Autodesk Inventor part; units mm, degrees
(part 5 of 5)
  line L348 (1.6512, 10.8975) -> (1.3983, 10.8975)
  line L349 (1.3983, 10.8975) -> (1.3983, 8.8084)
  line L350 (1.3983, 8.8084) -> (1.6512, 8.8084)
  line L351 (0.891, 9.7257) -> (0.0985, 9.7257)
  line L352 (1.1098, 8.9008) -> (1.1098, 9.1763)
  line L353 (1.1098, 9.1763) -> (1.0953, 9.1763)
  line L354 (0.0985, 9.5329) -> (1.1374, 9.5329)
  line L355 (1.1374, 9.5329) -> (1.1374, 9.6706)
  line L356 (-0.673, 10.0402) -> (-0.673, 9.1731)
  line L357 (-0.4201, 8.8084) -> (-0.4201, 10.8975)
  line L358 (-0.4201, 10.8975) -> (-0.673, 10.8975)
  line L359 (-0.673, 10.8975) -> (-0.673, 10.2492)
  line L360 (-0.673, 8.9607) -> (-0.673, 8.8084)
  line L361 (-0.673, 8.8084) -> (-0.4201, 8.8084)
  line L362 (-3.0409, 9.5944) -> (-3.0409, 9.1779)
  line L363 (-3.0409, 8.9672) -> (-3.0409, 8.8084)
  line L364 (-3.0409, 8.8084) -> (-2.7881, 8.8084)
  line L365 (-2.7881, 8.8084) -> (-2.7881, 9.8343)
  line L366 (-3.8626, 10.2768) -> (-3.8626, 10.0191)
  line L367 (-3.8626, 10.0191) -> (-3.848, 10.0191)
  line L368 (-3.0409, 9.844) -> (-3.0409, 9.7954)
  line L369 (-5.4996, 10.5588) -> (-5.4996, 10.8214)
  line L370 (-5.4996, 10.8214) -> (-5.7864, 10.8214)
  line L371 (-5.7864, 10.8214) -> (-5.7864, 10.5588)
  line L372 (-5.7864, 10.5588) -> (-5.4996, 10.5588)
  line L373 (-6.13, 8.8084) -> (-6.13, 9.7825)
  line L374 (-7.0555, 10.1423) -> (-7.0555, 10.3092)
  line L375 (-7.0555, 10.3092) -> (-7.3083, 10.3092)
  line L376 (-7.3083, 10.3092) -> (-7.3083, 8.8084)
  line L377 (-7.3083, 8.8084) -> (-7.0555, 8.8084)
  line L378 (-7.0555, 8.8084) -> (-7.0555, 9.9299)
  line L379 (-6.3829, 9.6641) -> (-6.3829, 8.8084)
  line L380 (-6.3829, 8.8084) -> (-6.13, 8.8084)
  line L381 (-7.9161, 9.5944) -> (-7.9161, 9.1779)
  line L382 (-7.9161, 8.9672) -> (-7.9161, 8.8084)
  line L383 (-7.9161, 8.8084) -> (-7.6633, 8.8084)
  line L384 (-7.6633, 8.8084) -> (-7.6633, 9.8343)
  line L385 (-8.7378, 10.2768) -> (-8.7378, 10.0191)
  line L386 (-8.7378, 10.0191) -> (-8.7232, 10.0191)
  line L387 (-7.9161, 9.844) -> (-7.9161, 9.7954)
  line L388 (-10.2516, 8.8927) -> (-10.2516, 9.1763)
  line L389 (-10.2516, 9.1763) -> (-10.2662, 9.1763)
  line L390 (-10.2662, 9.9445) -> (-10.2516, 9.9445)
  line L391 (-10.2516, 9.9445) -> (-10.2516, 10.2282)
  line L392 (-11.7929, 9.7257) -> (-12.5855, 9.7257)
  line L393 (-11.5741, 8.9008) -> (-11.5741, 9.1763)
  line L394 (-11.5741, 9.1763) -> (-11.5887, 9.1763)
  line L395 (-12.5855, 9.5329) -> (-11.5466, 9.5329)
  line L396 (-11.5466, 9.5329) -> (-11.5466, 9.6706)
  line L397 (-16.2597, 10.5588) -> (-16.2597, 10.8214)
  line L398 (-16.2597, 10.8214) -> (-16.5466, 10.8214)
  line L399 (-16.5466, 10.8214) -> (-16.5466, 10.5588)
  line L400 (-16.5466, 10.5588) -> (-16.2597, 10.5588)
  line L401 (-20.5936, 8.8214) -> (-20.5936, 9.0483)
  line L402 (-20.5936, 9.0483) -> (-20.6081, 9.0483)
  line L403 (-21.0587, 9.3854) -> (-21.0587, 10.1001)
  line L404 (-21.0587, 10.1001) -> (-20.5936, 10.1001)
  line L405 (-20.5936, 10.1001) -> (-20.5936, 10.3092)
  line L406 (-20.5936, 10.3092) -> (-21.0587, 10.3092)
  line L407 (-21.0587, 10.3092) -> (-21.0587, 10.7403)
  line L408 (-21.0587, 10.7403) -> (-21.3116, 10.7403)
  line L409 (-21.3116, 10.7403) -> (-21.3116, 10.3092)
  line L410 (-21.3116, 10.3092) -> (-21.4817, 10.3092)
  line L411 (-21.4817, 10.3092) -> (-21.4817, 10.1001)
  line L412 (-21.4817, 10.1001) -> (-21.3116, 10.1001)
  line L413 (-21.3116, 10.1001) -> (-21.3116, 9.2687)
  line L414 (-26.9047, 10.0385) -> (-26.9047, 10.3011)
  line L415 (-27.4477, 10.0855) -> (-27.4477, 10.3092)
  line L416 (-27.4477, 10.3092) -> (-27.7005, 10.3092)
  line L417 (-27.7005, 10.3092) -> (-27.7005, 8.8084)
  line L418 (-27.7005, 8.8084) -> (-27.4477, 8.8084)
  line L419 (-27.4477, 8.8084) -> (-27.4477, 9.8732)
  line L420 (-26.9177, 10.0385) -> (-26.9047, 10.0385)
  line L421 (-28.7508, 9.7808) -> (-28.9323, 9.7808)
  line L422 (-28.9323, 9.7808) -> (-28.9323, 10.5782)
  line L423 (-28.9323, 10.5782) -> (-28.7119, 10.5782)
  line L424 (-28.6957, 10.8084) -> (-29.1981, 10.8084)
  line L425 (-29.1981, 10.8084) -> (-29.1981, 8.8084)
  line L426 (-29.1981, 8.8084) -> (-28.9323, 8.8084)
  line L427 (-28.9323, 8.8084) -> (-28.9323, 9.5539)
  line L428 (-28.9323, 9.5539) -> (-28.707, 9.5539)
  line L429 (-24.3148, 10.0402) -> (-24.3148, 9.2152)
  line L430 (-25.1624, 8.5685) -> (-25.1754, 8.5685)
  line L431 (-25.1754, 8.5685) -> (-25.1754, 8.306)
  line L432 (-24.062, 8.9802) -> (-24.062, 10.3092)
  line L433 (-24.062, 10.3092) -> (-24.3002, 10.3092)
  line L434 (-24.3002, 10.3092) -> (-24.3148, 10.246)
  line L435 (-24.3148, 9.0077) -> (-24.3148, 8.8765)
  line L436 (-22.7508, 9.7257) -> (-23.5433, 9.7257)
  line L437 (-22.532, 8.9008) -> (-22.532, 9.1763)
  line L438 (-22.532, 9.1763) -> (-22.5466, 9.1763)
  line L439 (-23.5433, 9.5329) -> (-22.5044, 9.5329)
  line L440 (-22.5044, 9.5329) -> (-22.5044, 9.6706)
  line L441 (-21.5141, 8.8214) -> (-21.5141, 9.0483)
  line L442 (-21.5141, 9.0483) -> (-21.5287, 9.0483)
  line L443 (-21.9793, 9.3854) -> (-21.9793, 10.1001)
  line L444 (-21.9793, 10.1001) -> (-21.5141, 10.1001)
  line L445 (-21.5141, 10.1001) -> (-21.5141, 10.3092)
  line L446 (-21.5141, 10.3092) -> (-21.9793, 10.3092)
  line L447 (-21.9793, 10.3092) -> (-21.9793, 10.7403)
  line L448 (-21.9793, 10.7403) -> (-22.2321, 10.7403)
  line L449 (-22.2321, 10.7403) -> (-22.2321, 10.3092)
  line L450 (-22.2321, 10.3092) -> (-22.4023, 10.3092)
  line L451 (-22.4023, 10.3092) -> (-22.4023, 10.1001)
  line L452 (-22.4023, 10.1001) -> (-22.2321, 10.1001)
  line L453 (-22.2321, 10.1001) -> (-22.2321, 9.2687)
  line L454 (-17.1543, 10.0402) -> (-17.1543, 9.1731)
  line L455 (-16.9015, 8.8084) -> (-16.9015, 10.8975)
  line L456 (-16.9015, 10.8975) -> (-17.1543, 10.8975)
  line L457 (-17.1543, 10.8975) -> (-17.1543, 10.2492)
  line L458 (-17.1543, 8.9607) -> (-17.1543, 8.8084)
  line L459 (-17.1543, 8.8084) -> (-16.9015, 8.8084)
  line L460 (-16.2775, 8.8084) -> (-16.2775, 10.3092)
  line L461 (-16.2775, 10.3092) -> (-16.5304, 10.3092)
  line L462 (-16.5304, 10.3092) -> (-16.5304, 8.8084)
  line L463 (-16.5304, 8.8084) -> (-16.2775, 8.8084)
  line L464 (-13.3456, 8.8084) -> (-13.0928, 8.8084)
  line L465 (-13.0928, 8.8084) -> (-13.0928, 9.797)
  line L466 (-14.7945, 10.1439) -> (-14.7945, 10.3092)
  line L467 (-14.7945, 10.3092) -> (-15.0474, 10.3092)
  line L468 (-15.0474, 10.3092) -> (-15.0474, 8.8084)
  line L469 (-15.0474, 8.8084) -> (-14.7945, 8.8084)
  line L470 (-14.7945, 8.8084) -> (-14.7945, 9.9299)
  line L471 (-14.1965, 9.6771) -> (-14.1965, 8.8084)
  line L472 (-14.1965, 8.8084) -> (-13.9436, 8.8084)
  line L473 (-13.9436, 8.8084) -> (-13.9436, 9.797)
  line L474 (-13.3456, 9.6771) -> (-13.3456, 8.8084)
  line L475 (-8.9825, 8.8927) -> (-8.9825, 9.1763)
  line L476 (-8.9825, 9.1763) -> (-8.9971, 9.1763)
  line L477 (-8.9971, 9.9445) -> (-8.9825, 9.9445)
  line L478 (-8.9825, 9.9445) -> (-8.9825, 10.2282)
  line L479 (-5.5174, 8.8084) -> (-5.5174, 10.3092)
  line L480 (-5.5174, 10.3092) -> (-5.7702, 10.3092)
  line L481 (-5.7702, 10.3092) -> (-5.7702, 8.8084)
  line L482 (-5.7702, 8.8084) -> (-5.5174, 8.8084)
  line L483 (-4.1073, 8.8927) -> (-4.1073, 9.1763)
  line L484 (-4.1073, 9.1763) -> (-4.1219, 9.1763)
  line L485 (-4.1219, 9.9445) -> (-4.1073, 9.9445)
  line L486 (-4.1073, 9.9445) -> (-4.1073, 10.2282)
  line L487 (2.28, 8.8084) -> (2.28, 10.8975)
  line L488 (2.28, 10.8975) -> (2.0272, 10.8975)
  line L489 (2.0272, 10.8975) -> (2.0272, 8.8084)
  line L490 (2.0272, 8.8084) -> (2.28, 8.8084)
  line L491 (6.5847, 8.8084) -> (6.5847, 10.3092)
  line L492 (6.5847, 10.3092) -> (6.3319, 10.3092)
  line L493 (6.3319, 10.3092) -> (6.3319, 8.8084)
  line L494 (6.3319, 8.8084) -> (6.5847, 8.8084)
  line L495 (7.2087, 9.079) -> (7.2087, 9.9397)
  line L496 (7.2087, 10.152) -> (7.2087, 10.8975)
  line L497 (7.2087, 10.8975) -> (6.9559, 10.8975)
  line L498 (6.9559, 10.8975) -> (6.9559, 8.8084)
  line L499 (6.9559, 8.8084) -> (7.1925, 8.8084)
  line L500 (7.1925, 8.8084) -> (7.2087, 8.8781)
  line L501 (9.2719, 10.0385) -> (9.2719, 10.3011)
  line L502 (8.729, 10.0855) -> (8.729, 10.3092)
  line L503 (8.729, 10.3092) -> (8.4761, 10.3092)
  line L504 (8.4761, 10.3092) -> (8.4761, 8.8084)
  line L505 (8.4761, 8.8084) -> (8.729, 8.8084)
  line L506 (8.729, 8.8084) -> (8.729, 9.8732)
  line L507 (9.2589, 10.0385) -> (9.2719, 10.0385)
  line L508 (12.3919, 8.8084) -> (12.3919, 10.3092)
  line L509 (12.3919, 10.3092) -> (12.139, 10.3092)
  line L510 (12.139, 10.3092) -> (12.139, 8.8084)
  line L511 (12.139, 8.8084) -> (12.3919, 8.8084)
  line L512 (15.434, 8.8084) -> (15.434, 9.7825)
  line L513 (14.5085, 10.1423) -> (14.5085, 10.3092)
  line L514 (14.5085, 10.3092) -> (14.2557, 10.3092)
  line L515 (14.2557, 10.3092) -> (14.2557, 8.8084)
  line L516 (14.2557, 8.8084) -> (14.5085, 8.8084)
  line L517 (14.5085, 8.8084) -> (14.5085, 9.9299)
  line L518 (15.1812, 9.6641) -> (15.1812, 8.8084)
  line L519 (15.1812, 8.8084) -> (15.434, 8.8084)
  line L520 (16.0645, 10.5588) -> (16.0645, 10.8214)
  line L521 (16.0645, 10.8214) -> (15.7776, 10.8214)
  line L522 (15.7776, 10.8214) -> (15.7776, 10.5588)
  line L523 (15.7776, 10.5588) -> (16.0645, 10.5588)
  line L524 (21.374, 8.8084) -> (21.374, 9.0126)
  line L525 (21.374, 9.0126) -> (21.0191, 9.0126)
  line L526 (21.0191, 9.0126) -> (21.0191, 10.8149)
  line L527 (21.0191, 10.8149) -> (20.8116, 10.8149)
  line L528 (20.3983, 10.5361) -> (20.3983, 10.353)
  line L529 (20.3983, 10.353) -> (20.7614, 10.353)
  line L530 (20.7614, 10.353) -> (20.7614, 9.0126)
  line L531 (20.7614, 9.0126) -> (20.3983, 9.0126)
  line L532 (20.3983, 9.0126) -> (20.3983, 8.8084)
  line L533 (20.3983, 8.8084) -> (21.374, 8.8084)
  line L534 (25.528, 8.8084) -> (25.528, 9.0402)
  line L535 (25.528, 9.0402) -> (24.5458, 9.0402)
  line L536 (24.3367, 10.7306) -> (24.3367, 10.4453)
  line L537 (24.3367, 10.4453) -> (24.3513, 10.4453)
  line L538 (24.2946, 9.092) -> (24.2946, 8.8084)
  line L539 (24.2946, 8.8084) -> (25.528, 8.8084)
  line L540 (-26.7605, 6.3015) -> (-26.7605, 5.885)
  line L541 (-26.7605, 5.6743) -> (-26.7605, 5.5154)
  line L542 (-26.7605, 5.5154) -> (-26.5077, 5.5154)
  line L543 (-26.5077, 5.5154) -> (-26.5077, 6.5414)
  line L544 (-27.5822, 6.9838) -> (-27.5822, 6.7261)
  line L545 (-27.5822, 6.7261) -> (-27.5676, 6.7261)
  line L546 (-26.7605, 6.5511) -> (-26.7605, 6.5025)
  line L547 (-24.9744, 5.5154) -> (-24.9744, 6.4895)
  line L548 (-25.8999, 6.8493) -> (-25.8999, 7.0162)
  line L549 (-25.8999, 7.0162) -> (-26.1527, 7.0162)
  line L550 (-26.1527, 7.0162) -> (-26.1527, 5.5154)
  line L551 (-26.1527, 5.5154) -> (-25.8999, 5.5154)
  line L552 (-25.8999, 5.5154) -> (-25.8999, 6.637)
  line L553 (-25.2273, 6.3712) -> (-25.2273, 5.5154)
  line L554 (-25.2273, 5.5154) -> (-24.9744, 5.5154)
  line L555 (-20.0976, 6.7472) -> (-20.0976, 5.8801)
  line L556 (-19.8448, 5.5154) -> (-19.8448, 7.6046)
  line L557 (-19.8448, 7.6046) -> (-20.0976, 7.6046)
  line L558 (-20.0976, 7.6046) -> (-20.0976, 6.9563)
  line L559 (-20.0976, 5.6678) -> (-20.0976, 5.5154)
  line L560 (-20.0976, 5.5154) -> (-19.8448, 5.5154)
  line L561 (-19.2208, 5.5154) -> (-19.2208, 7.0162)
  line L562 (-19.2208, 7.0162) -> (-19.4736, 7.0162)
  line L563 (-19.4736, 7.0162) -> (-19.4736, 5.5154)
  line L564 (-19.4736, 5.5154) -> (-19.2208, 5.5154)
  line L565 (-17.7378, 5.7958) -> (-17.7378, 6.6483)
  line L566 (-17.7378, 6.859) -> (-17.7378, 7.0162)
  line L567 (-17.7378, 7.0162) -> (-17.9906, 7.0162)
  line L568 (-17.9906, 7.0162) -> (-17.9906, 4.9628)
  line L569 (-17.9906, 4.9628) -> (-17.7378, 4.9628)
  line L570 (-17.7378, 4.9628) -> (-17.7378, 5.5916)
  line L571 (-15.6746, 6.7456) -> (-15.6746, 7.0081)
  line L572 (-16.2175, 6.7926) -> (-16.2175, 7.0162)
  line L573 (-16.2175, 7.0162) -> (-16.4704, 7.0162)
  line L574 (-16.4704, 7.0162) -> (-16.4704, 5.5154)
  line L575 (-16.4704, 5.5154) -> (-16.2175, 5.5154)
  line L576 (-16.2175, 5.5154) -> (-16.2175, 6.5803)
  line L577 (-15.6876, 6.7456) -> (-15.6746, 6.7456)
  line L578 (-11.7799, 6.3015) -> (-11.7799, 5.885)
  line L579 (-11.7799, 5.6743) -> (-11.7799, 5.5154)
  line L580 (-11.7799, 5.5154) -> (-11.5271, 5.5154)
  line L581 (-11.5271, 5.5154) -> (-11.5271, 6.5414)
  line L582 (-12.6017, 6.9838) -> (-12.6017, 6.7261)
  line L583 (-12.6017, 6.7261) -> (-12.5871, 6.7261)
  line L584 (-11.7799, 6.5511) -> (-11.7799, 6.5025)
  line L585 (-10.0603, 5.7958) -> (-10.0603, 6.6483)
  line L586 (-10.0603, 6.859) -> (-10.0603, 7.0162)
  line L587 (-10.0603, 7.0162) -> (-10.3132, 7.0162)
  line L588 (-10.3132, 7.0162) -> (-10.3132, 4.9628)
  line L589 (-10.3132, 4.9628) -> (-10.0603, 4.9628)
  line L590 (-10.0603, 4.9628) -> (-10.0603, 5.5916)
  line L591 (-7.848, 6.4328) -> (-8.6406, 6.4328)
  line L592 (-7.6292, 5.6078) -> (-7.6292, 5.8833)
  line L593 (-7.6292, 5.8833) -> (-7.6438, 5.8833)
  line L594 (-8.6406, 6.2399) -> (-7.6017, 6.2399)
  line L595 (-7.6017, 6.2399) -> (-7.6017, 6.3777)
  line L596 (-6.5498, 6.7456) -> (-6.5498, 7.0081)
  line L597 (-7.0928, 6.7926) -> (-7.0928, 7.0162)
  line L598 (-7.0928, 7.0162) -> (-7.3456, 7.0162)
  line L599 (-7.3456, 7.0162) -> (-7.3456, 5.5154)
  line L600 (-7.3456, 5.5154) -> (-7.0928, 5.5154)
  line L601 (-7.0928, 5.5154) -> (-7.0928, 6.5803)
  line L602 (-6.5628, 6.7456) -> (-6.5498, 6.7456)
  line L603 (-0.9582, 5.5284) -> (-0.9582, 5.7553)
  line L604 (-0.9582, 5.7553) -> (-0.9728, 5.7553)
  line L605 (-1.4234, 6.0924) -> (-1.4234, 6.8072)
  line L606 (-1.4234, 6.8072) -> (-0.9582, 6.8072)
  line L607 (-0.9582, 6.8072) -> (-0.9582, 7.0162)
  line L608 (-0.9582, 7.0162) -> (-1.4234, 7.0162)
  line L609 (-1.4234, 7.0162) -> (-1.4234, 7.4474)
  line L610 (-1.4234, 7.4474) -> (-1.6762, 7.4474)
  line L611 (-1.6762, 7.4474) -> (-1.6762, 7.0162)
  line L612 (-1.6762, 7.0162) -> (-1.8464, 7.0162)
  line L613 (-1.8464, 7.0162) -> (-1.8464, 6.8072)
  line L614 (-1.8464, 6.8072) -> (-1.6762, 6.8072)
  line L615 (-1.6762, 6.8072) -> (-1.6762, 5.9757)
  line L616 (2.6577, 6.4328) -> (1.8651, 6.4328)
  line L617 (2.8765, 5.6078) -> (2.8765, 5.8833)
  line L618 (2.8765, 5.8833) -> (2.8619, 5.8833)
  line L619 (1.8651, 6.2399) -> (2.904, 6.2399)
  line L620 (2.904, 6.2399) -> (2.904, 6.3777)
  line L621 (4.5069, 5.7456) -> (4.3043, 5.7456)
  line L622 (4.3043, 5.7456) -> (4.3043, 7.2853)
  line L623 (4.3043, 7.2853) -> (4.5069, 7.2853)
  line L624 (4.494, 7.5154) -> (4.0385, 7.5154)
  line L625 (4.0385, 7.5154) -> (4.0385, 5.5154)
  line L626 (4.0385, 5.5154) -> (4.4988, 5.5154)
  line L627 (7.3076, 5.6516) -> (7.3076, 5.9692)
  line L628 (7.3076, 5.9692) -> (7.2881, 5.9692)
  line L629 (7.2865, 7.0616) -> (7.3076, 7.0616)
  line L630 (7.3076, 7.0616) -> (7.3076, 7.3825)
  line L631 (-24.2727, 2.2225) -> (-24.2727, 3.7233)
  line L632 (-24.2727, 3.7233) -> (-24.5255, 3.7233)
  line L633 (-24.5255, 3.7233) -> (-24.5255, 2.6017)
  line L634 (-25.1981, 2.8675) -> (-25.1981, 3.7233)
  line L635 (-25.1981, 3.7233) -> (-25.4509, 3.7233)
  line L636 (-25.4509, 3.7233) -> (-25.4509, 2.7492)
  line L637 (-24.5255, 2.3878) -> (-24.5255, 2.2225)
  line L638 (-24.5255, 2.2225) -> (-24.2727, 2.2225)
  line L639 (-22.0782, 3.0086) -> (-22.0782, 2.592)
  line L640 (-22.0782, 2.3813) -> (-22.0782, 2.2225)
  line L641 (-22.0782, 2.2225) -> (-21.8253, 2.2225)
  line L642 (-21.8253, 2.2225) -> (-21.8253, 3.2484)
  line L643 (-22.8999, 3.6909) -> (-22.8999, 3.4332)
  line L644 (-22.8999, 3.4332) -> (-22.8853, 3.4332)
  line L645 (-22.0782, 3.2581) -> (-22.0782, 3.2095)
  line L646 (-19.7103, 3.4543) -> (-19.7103, 2.5872)
  line L647 (-19.4574, 2.2225) -> (-19.4574, 4.3116)
  line L648 (-19.4574, 4.3116) -> (-19.7103, 4.3116)
  line L649 (-19.7103, 4.3116) -> (-19.7103, 3.6633)
  line L650 (-19.7103, 2.3748) -> (-19.7103, 2.2225)
  line L651 (-19.7103, 2.2225) -> (-19.4574, 2.2225)
  line L652 (-18.8334, 2.2225) -> (-18.8334, 3.7233)
  line L653 (-18.8334, 3.7233) -> (-19.0863, 3.7233)
  line L654 (-19.0863, 3.7233) -> (-19.0863, 2.2225)
  line L655 (-19.0863, 2.2225) -> (-18.8334, 2.2225)
  line L656 (-17.9987, 2.2225) -> (-17.9987, 2.605)
  line L657 (-17.9987, 2.605) -> (-18.3197, 2.605)
  line L658 (-18.3197, 2.605) -> (-18.3197, 2.2225)
  line L659 (-18.3197, 2.2225) -> (-17.9987, 2.2225)
  line L660 (-20.1495, 0.7756) -> (-20.1495, 1.0073)
  line L661 (-20.9128, 0.4806) -> (-20.9128, 0.4304)
  line L662 (-20.9128, 0.4304) -> (-21.083, 0.4304)
  line L663 (-21.083, 0.4304) -> (-21.083, 0.2213)
  line L664 (-21.083, 0.2213) -> (-20.9128, 0.2213)
  line L665 (-20.9128, 0.2213) -> (-20.9128, -1.0705)
  line L666 (-20.9128, -1.0705) -> (-20.66, -1.0705)
  line L667 (-20.66, -1.0705) -> (-20.66, 0.2213)
  line L668 (-20.66, 0.2213) -> (-20.25, 0.2213)
  line L669 (-20.25, 0.2213) -> (-20.25, 0.4304)
  line L670 (-20.25, 0.4304) -> (-20.6681, 0.4304)
  line L671 (-20.6681, 0.4304) -> (-20.6681, 0.4806)
  line L672 (-20.1624, 0.7756) -> (-20.1495, 0.7756)
  line L673 (-14.7151, -1.0705) -> (-13.4639, -1.0705)
  line L674 (-13.4639, -1.0705) -> (-13.4639, -0.8338)
  line L675 (-13.4639, -0.8338) -> (-14.4493, -0.8338)
  line L676 (-14.4493, -0.8338) -> (-14.4493, -0.0915)
  line L677 (-14.4493, -0.0915) -> (-13.5304, -0.0915)
  line L678 (-13.5304, -0.0915) -> (-13.5304, 0.1451)
  line L679 (-13.5304, 0.1451) -> (-14.4493, 0.1451)
  line L680 (-14.4493, 0.1451) -> (-14.4493, 0.6929)
  line L681 (-14.4493, 0.6929) -> (-13.4639, 0.6929)
  line L682 (-13.4639, 0.6929) -> (-13.4639, 0.9295)
  line L683 (-13.4639, 0.9295) -> (-14.7151, 0.9295)
  line L684 (-14.7151, 0.9295) -> (-14.7151, -1.0705)
  line L685 (-10.0458, -0.2844) -> (-10.0458, -0.7009)
  line L686 (-10.0458, -0.9116) -> (-10.0458, -1.0705)
  line L687 (-10.0458, -1.0705) -> (-9.7929, -1.0705)
  line L688 (-9.7929, -1.0705) -> (-9.7929, -0.0445)
  line L689 (-10.8675, 0.3979) -> (-10.8675, 0.1402)
  line L690 (-10.8675, 0.1402) -> (-10.8529, 0.1402)
  line L691 (-10.0458, -0.0348) -> (-10.0458, -0.0834)
  line L692 (-8.2597, -1.0705) -> (-8.2597, -0.0964)
  line L693 (-9.1851, 0.2634) -> (-9.1851, 0.4304)
  line L694 (-9.1851, 0.4304) -> (-9.438, 0.4304)
  line L695 (-9.438, 0.4304) -> (-9.438, -1.0705)
  line L696 (-9.438, -1.0705) -> (-9.1851, -1.0705)
  line L697 (-9.1851, -1.0705) -> (-9.1851, 0.0511)
  line L698 (-8.5125, -0.2147) -> (-8.5125, -1.0705)
  line L699 (-8.5125, -1.0705) -> (-8.2597, -1.0705)
  line L700 (-5.4266, -0.1531) -> (-6.2192, -0.1531)
  line L701 (-5.2078, -0.9781) -> (-5.2078, -0.7025)
  line L702 (-5.2078, -0.7025) -> (-5.2224, -0.7025)
  line L703 (-6.2192, -0.346) -> (-5.1803, -0.346)
  line L704 (-5.1803, -0.346) -> (-5.1803, -0.2082)
  line L705 (-4.6665, -1.0705) -> (-4.6665, 1.0187)
  line L706 (-4.6665, 1.0187) -> (-4.9193, 1.0187)
  line L707 (-4.9193, 1.0187) -> (-4.9193, -1.0705)
  line L708 (-4.9193, -1.0705) -> (-4.6665, -1.0705)
  line L709 (-22.6308, -3.1754) -> (-22.9323, -3.1754)
  line L710 (-22.9323, -3.1754) -> (-22.9323, -2.5903)
  line L711 (-22.9323, -2.5903) -> (-22.6778, -2.5903)
  line L712 (-22.7167, -4.1365) -> (-22.9323, -4.1365)
  line L713 (-22.9323, -4.1365) -> (-22.9323, -3.3974)
  line L714 (-22.9323, -3.3974) -> (-22.6308, -3.3974)
  line L715 (-22.2159, -3.2516) -> (-22.2159, -3.2418)
  line L716 (-22.6681, -2.3634) -> (-23.1981, -2.3634)
  line L717 (-23.1981, -2.3634) -> (-23.1981, -4.3634)
  line L718 (-23.1981, -4.3634) -> (-22.6244, -4.3634)
  line L719 (-15.7232, -3.5773) -> (-15.7232, -3.9939)
  line L720 (-15.7232, -4.2046) -> (-15.7232, -4.3634)
  line L721 (-15.7232, -4.3634) -> (-15.4704, -4.3634)
  line L722 (-15.4704, -4.3634) -> (-15.4704, -3.3375)
  line L723 (-16.5449, -2.895) -> (-16.5449, -3.1527)
  line L724 (-16.5449, -3.1527) -> (-16.5304, -3.1527)
  line L725 (-15.7232, -3.3277) -> (-15.7232, -3.3764)
  line L726 (-13.4137, -4.3634) -> (-13.1608, -4.3634)
  line L727 (-13.1608, -4.3634) -> (-13.1608, -3.3747)
  line L728 (-14.8626, -3.0279) -> (-14.8626, -2.8626)
  line L729 (-14.8626, -2.8626) -> (-15.1154, -2.8626)
  line L730 (-15.1154, -2.8626) -> (-15.1154, -4.3634)
  line L731 (-15.1154, -4.3634) -> (-14.8626, -4.3634)
  line L732 (-14.8626, -4.3634) -> (-14.8626, -3.2418)
  line L733 (-14.2646, -3.4947) -> (-14.2646, -4.3634)
  line L734 (-14.2646, -4.3634) -> (-14.0117, -4.3634)
  line L735 (-14.0117, -4.3634) -> (-14.0117, -3.3747)
  line L736 (-13.4137, -3.4947) -> (-13.4137, -4.3634)
  line L737 (-9.0911, -4.3504) -> (-9.0911, -4.1235)
  line L738 (-9.0911, -4.1235) -> (-9.1057, -4.1235)
  line L739 (-9.5563, -3.7864) -> (-9.5563, -3.0717)
  line L740 (-9.5563, -3.0717) -> (-9.0911, -3.0717)
  line L741 (-9.0911, -3.0717) -> (-9.0911, -2.8626)
  line L742 (-9.0911, -2.8626) -> (-9.5563, -2.8626)
  line L743 (-9.5563, -2.8626) -> (-9.5563, -2.4315)
  line L744 (-9.5563, -2.4315) -> (-9.8091, -2.4315)
  line L745 (-9.8091, -2.4315) -> (-9.8091, -2.8626)
  line L746 (-9.8091, -2.8626) -> (-9.9793, -2.8626)
  line L747 (-9.9793, -2.8626) -> (-9.9793, -3.0717)
  line L748 (-9.9793, -3.0717) -> (-9.8091, -3.0717)
  line L749 (-9.8091, -3.0717) -> (-9.8091, -3.9031)
  line L750 (-8.6292, -2.613) -> (-8.6292, -2.3504)
  line L751 (-8.6292, -2.3504) -> (-8.9161, -2.3504)
  line L752 (-8.9161, -2.3504) -> (-8.9161, -2.613)
  line L753 (-8.9161, -2.613) -> (-8.6292, -2.613)
  line L754 (-5.7248, -4.3634) -> (-5.7248, -2.8626)
  line L755 (-5.7248, -2.8626) -> (-5.9777, -2.8626)
  line L756 (-5.9777, -2.8626) -> (-5.9777, -4.3634)
  line L757 (-5.9777, -4.3634) -> (-5.7248, -4.3634)
  line L758 (-5.096, -4.3634) -> (-5.096, -2.2743)
  line L759 (-5.096, -2.2743) -> (-5.3488, -2.2743)
  line L760 (-5.3488, -2.2743) -> (-5.3488, -4.3634)
  line L761 (-5.3488, -4.3634) -> (-5.096, -4.3634)
  line L762 (-4.4493, -2.613) -> (-4.4493, -2.3504)
  line L763 (-4.4493, -2.3504) -> (-4.7362, -2.3504)
  line L764 (-4.7362, -2.3504) -> (-4.7362, -2.613)
  line L765 (-4.7362, -2.613) -> (-4.4493, -2.613)
  line L766 (-21.7475, -5.6564) -> (-22.0182, -5.6564)
  line L767 (-22.0182, -5.6564) -> (-22.5725, -7.3176)
  line L768 (-22.5725, -7.3176) -> (-23.1268, -5.6564)
  line L769 (-23.1268, -5.6564) -> (-23.412, -5.6564)
  line L770 (-23.412, -5.6564) -> (-22.7232, -7.6564)
  line L771 (-22.7232, -7.6564) -> (-22.4364, -7.6564)
  line L772 (-22.4364, -7.6564) -> (-21.7475, -5.6564)
  line L773 (-21.3002, -5.9059) -> (-21.3002, -5.6434)
  line L774 (-21.3002, -5.6434) -> (-21.5871, -5.6434)
  line L775 (-21.5871, -5.6434) -> (-21.5871, -5.9059)
  line L776 (-21.5871, -5.9059) -> (-21.3002, -5.9059)
  line L777 (-19.2921, -7.6434) -> (-19.2921, -7.4165)
  line L778 (-19.2921, -7.4165) -> (-19.3067, -7.4165)
  line L779 (-19.7573, -7.0794) -> (-19.7573, -6.3646)
  line L780 (-19.7573, -6.3646) -> (-19.2921, -6.3646)
  line L781 (-19.2921, -6.3646) -> (-19.2921, -6.1555)
  line L782 (-19.2921, -6.1555) -> (-19.7573, -6.1555)
  line L783 (-19.7573, -6.1555) -> (-19.7573, -5.7244)
  line L784 (-19.7573, -5.7244) -> (-20.0101, -5.7244)
  line L785 (-20.0101, -5.7244) -> (-20.0101, -6.1555)
  line L786 (-20.0101, -6.1555) -> (-20.1803, -6.1555)
  line L787 (-20.1803, -6.1555) -> (-20.1803, -6.3646)
  line L788 (-20.1803, -6.3646) -> (-20.0101, -6.3646)
  line L789 (-20.0101, -6.3646) -> (-20.0101, -7.1961)
  line L790 (-18.8302, -5.9059) -> (-18.8302, -5.6434)
  line L791 (-18.8302, -5.6434) -> (-19.1171, -5.6434)
  line L792 (-19.1171, -5.6434) -> (-19.1171, -5.9059)
  line L793 (-19.1171, -5.9059) -> (-18.8302, -5.9059)
  line L794 (-14.9453, -6.8703) -> (-14.9453, -7.2868)
  line L795 (-14.9453, -7.4975) -> (-14.9453, -7.6564)
  line L796 (-14.9453, -7.6564) -> (-14.6924, -7.6564)
  line L797 (-14.6924, -7.6564) -> (-14.6924, -6.6304)
  line L798 (-15.767, -6.188) -> (-15.767, -6.4457)
  line L799 (-15.767, -6.4457) -> (-15.7524, -6.4457)
  line L800 (-14.9453, -6.6207) -> (-14.9453, -6.6693)
  line L801 (-14.0846, -7.3857) -> (-14.0846, -6.5251)
  line L802 (-14.0846, -6.3128) -> (-14.0846, -5.5672)
  line L803 (-14.0846, -5.5672) -> (-14.3375, -5.5672)
  line L804 (-14.3375, -5.5672) -> (-14.3375, -7.6564)
  line L805 (-14.3375, -7.6564) -> (-14.1009, -7.6564)
  line L806 (-14.1009, -7.6564) -> (-14.0846, -7.5867)
  line L807 (-12.0214, -6.4262) -> (-12.0214, -6.1636)
  line L808 (-12.5644, -6.3792) -> (-12.5644, -6.1555)
  line L809 (-12.5644, -6.1555) -> (-12.8172, -6.1555)
  line L810 (-12.8172, -6.1555) -> (-12.8172, -7.6564)
  line L811 (-12.8172, -7.6564) -> (-12.5644, -7.6564)
  line L812 (-12.5644, -7.6564) -> (-12.5644, -6.5915)
  line L813 (-12.0344, -6.4262) -> (-12.0214, -6.4262)
  line L814 (-11.5498, -5.9059) -> (-11.5498, -5.6434)
  line L815 (-11.5498, -5.6434) -> (-11.8367, -5.6434)
  line L816 (-11.8367, -5.6434) -> (-11.8367, -5.9059)
  line L817 (-11.8367, -5.9059) -> (-11.5498, -5.9059)
  line L818 (-8.1754, -6.739) -> (-8.968, -6.739)
  line L819 (-7.9566, -7.564) -> (-7.9566, -7.2884)
  line L820 (-7.9566, -7.2884) -> (-7.9712, -7.2884)
  line L821 (-8.968, -6.9319) -> (-7.9291, -6.9319)
  line L822 (-7.9291, -6.9319) -> (-7.9291, -6.7941)
  line L823 (-19.1543, -10.865) -> (-19.1543, -10.5814)
  line L824 (-19.1543, -10.5814) -> (-19.1689, -10.5814)
  line L825 (-19.1689, -9.8132) -> (-19.1543, -9.8132)
  line L826 (-19.1543, -9.8132) -> (-19.1543, -9.5295)
  line L827 (-17.3975, -10.9493) -> (-17.3975, -9.4485)
  line L828 (-17.3975, -9.4485) -> (-17.6503, -9.4485)
  line L829 (-17.6503, -9.4485) -> (-17.6503, -10.9493)
  line L830 (-17.6503, -10.9493) -> (-17.3975, -10.9493)
  line L831 (-13.4963, -10.9493) -> (-13.4963, -10.7127)
  line L832 (-13.4963, -10.7127) -> (-14.3893, -10.7127)
  line L833 (-14.3893, -10.7127) -> (-14.3893, -8.9493)
  line L834 (-14.3893, -8.9493) -> (-14.6552, -8.9493)
  line L835 (-14.6552, -8.9493) -> (-14.6552, -10.9493)
  line L836 (-14.6552, -10.9493) -> (-13.4963, -10.9493)
  line L837 (-7.9971, -10.1632) -> (-7.9971, -10.5798)
  line L838 (-7.9971, -10.7905) -> (-7.9971, -10.9493)
  line L839 (-7.9971, -10.9493) -> (-7.7443, -10.9493)
  line L840 (-7.7443, -10.9493) -> (-7.7443, -9.9234)
  line L841 (-8.8188, -9.4809) -> (-8.8188, -9.7386)
  line L842 (-8.8188, -9.7386) -> (-8.8043, -9.7386)
  line L843 (-7.9971, -9.9136) -> (-7.9971, -9.9623)
  line L844 (-6.5936, -9.7192) -> (-6.5936, -9.4566)
  line L845 (-7.1365, -9.6722) -> (-7.1365, -9.4485)
  line L846 (-7.1365, -9.4485) -> (-7.3893, -9.4485)
  line L847 (-7.3893, -9.4485) -> (-7.3893, -10.9493)
  line L848 (-7.3893, -10.9493) -> (-7.1365, -10.9493)
  line L849 (-7.1365, -10.9493) -> (-7.1365, -9.8845)
  line L850 (-6.6065, -9.7192) -> (-6.5936, -9.7192)
  point P0 (0, 0)
  point P1 (-4.7232, -10.1989)
  point P2 (-4.3132, -9.6235)
  point P3 (-3.9047, -10.1989)
  point P4 (-4.3132, -10.7743)
  point P5 (-3.6438, -10.1989)
  point P6 (-4.3132, -9.4063)
  point P7 (-4.9842, -10.1989)
  point P8 (-4.3132, -10.9914)
  point P9 (-5.8253, -9.6381)
  point P10 (-5.8853, -10.7516)
  point P11 (-6.2402, -10.2054)
  point P12 (-5.8675, -9.4063)
  point P13 (-6.3099, -9.6154)
  point P14 (-6.5012, -10.2102)
  point P15 (-6.3472, -10.7905)
  point P16 (-5.9436, -10.9914)
  point P17 (-5.6989, -10.938)
  point P18 (-9.6584, -9.4063)
  point P19 (-9.7248, -9.6462)
  point P20 (-9.4898, -9.758)
  point P21 (-11.7054, -10.1989)
  point P22 (-11.2953, -9.6235)
  point P23 (-10.8869, -10.1989)
  point P24 (-11.2953, -10.7743)
  point P25 (-10.626, -10.1989)
  point P26 (-11.2953, -9.4063)
  point P27 (-11.9663, -10.1989)
  point P28 (-11.2953, -10.9914)
  point P29 (-12.7313, -9.6138)
  point P30 (-12.4477, -9.7305)
  point P31 (-13.0312, -9.7321)
  point P32 (-12.6552, -10.9833)
  point P33 (-12.3715, -10.9412)
  point P34 (-12.3505, -10.6965)
  point P35 (-12.6584, -10.7629)
  point P36 (-12.2824, -9.5733)
  point P37 (-12.7167, -9.4063)
  point P38 (-13.4104, -10.207)
  point P39 (-18.3278, -10.9833)
  point P40 (-18.0814, -10.9444)
  point P41 (-18.3326, -10.7629)
  point P42 (-18.767, -10.2021)
  point P43 (-18.3326, -9.6349)
  point P44 (-18.0717, -9.7013)
  point P45 (-18.3278, -9.4145)
  point P46 (-18.8334, -9.6187)
  point P47 (-19.0279, -10.2021)
  point P48 (-18.8334, -10.7905)
  point P49 (-22.6406, -10.985)
  point P50 (-22.1187, -10.8034)
  point P51 (-21.9372, -10.3788)
  point P52 (-22.3342, -9.8747)
  point P53 (-22.7443, -9.7694)
  point P54 (-23.0052, -9.4582)
  point P55 (-22.5919, -9.1438)
  point P56 (-22.6098, -8.9136)
  point P57 (-23.2824, -9.4858)
  point P58 (-23.1527, -9.8472)
  point P59 (-22.8221, -10.0239)
  point P60 (-22.4607, -10.1146)
  point P61 (-22.2143, -10.4209)
  point P62 (-22.66, -10.7548)
  point P63 (-10.6211, -6.3209)
  point P64 (-10.3375, -6.4376)
  point P65 (-10.921, -6.4392)
  point P66 (-10.5449, -7.6904)
  point P67 (-10.2613, -7.6482)
  point P68 (-10.2402, -7.4035)
  point P69 (-10.5482, -7.47)
  point P70 (-10.1722, -6.2803)
  point P71 (-10.6065, -6.1134)
  point P72 (-11.3002, -6.914)
  point P73 (-16.7605, -7.6952)
  point P74 (-16.391, -7.6369)
  point P75 (-16.7702, -7.4651)
  point P76 (-17.2516, -7.2528)
  point P77 (-17.4347, -6.6466)
  point P78 (-16.7897, -5.8508)
  point P79 (-16.3796, -5.9448)
  point P80 (-16.3877, -5.6758)
  point P81 (-16.7589, -5.6207)
  point P82 (-17.4493, -5.8946)
  point P83 (-17.7119, -6.6547)
  point P84 (-17.4509, -7.4343)
  point P85 (-20.4931, -7.6855)
  point P86 (-20.4299, -7.4651)
  point P87 (-20.6422, -7.3711)
  point P88 (-28.3034, -6.7682)
  point P89 (-28.7767, -6.2965)
  point P90 (-29.2483, -6.7682)
  point P91 (-28.7767, -7.2398)
  point P92 (-0.9015, -3.613)
  point P93 (-0.4915, -3.0376)
  point P94 (-0.083, -3.613)
  point P95 (-0.4915, -4.1884)
  point P96 (0.1779, -3.613)
  point P97 (-0.4915, -2.8205)
  point P98 (-1.1624, -3.613)
  point P99 (-0.4915, -4.4055)
  point P100 (-1.9258, -3.0603)
  point P101 (-1.579, -3.6017)
  point P102 (-1.9923, -4.1657)
  point P103 (-1.318, -3.5725)
  point P104 (-1.8642, -2.8205)
  point P105 (-1.9501, -4.3926)
  point P106 (-3.4461, -3.0603)
  point P107 (-3.0992, -3.6017)
  point P108 (-3.5125, -4.1657)
  point P109 (-2.8383, -3.5725)
  point P110 (-3.3845, -2.8205)
  point P111 (-3.4704, -4.3926)
  point P112 (-10.6503, -2.8205)
  point P113 (-10.7167, -3.0603)
  point P114 (-10.4817, -3.1722)
  point P115 (-12.2305, -3.0279)
  point P116 (-11.9469, -3.1446)
  point P117 (-12.5304, -3.1462)
  point P118 (-12.1543, -4.3974)
  point P119 (-11.8707, -4.3553)
  point P120 (-11.8496, -4.1106)
  point P121 (-12.1576, -4.177)
  point P122 (-11.7816, -2.9874)
  point P123 (-12.2159, -2.8205)
  point P124 (-12.9096, -3.6211)
  point P125 (-18.2467, -3.6389)
  point P126 (-18.1932, -4.1722)
  point P127 (-18.4785, -3.9112)
  point P128 (-17.707, -2.9388)
  point P129 (-18.1592, -2.8269)
  point P130 (-18.1608, -3.0506)
  point P131 (-17.8983, -3.1008)
  point P132 (-18.4655, -3.4898)
  point P133 (-18.7394, -3.929)
  point P134 (-18.6065, -4.2726)
  point P135 (-18.284, -4.4055)
  point P136 (-17.9793, -4.3326)
  point P137 (-19.5806, -3.0522)
  point P138 (-19.6406, -4.1657)
  point P139 (-19.9955, -3.6195)
  point P140 (-19.6227, -2.8205)
  point P141 (-20.0652, -3.0295)
  point P142 (-20.2564, -3.6243)
  point P143 (-20.1025, -4.2046)
  point P144 (-19.6989, -4.4055)
  point P145 (-19.4542, -4.3521)
  point P146 (-21.2111, -3.6389)
  point P147 (-21.1576, -4.1722)
  point P148 (-21.4428, -3.9112)
  point P149 (-20.6714, -2.9388)
  point P150 (-21.1235, -2.8269)
  point P151 (-21.1252, -3.0506)
  point P152 (-20.8626, -3.1008)
  point P153 (-21.4299, -3.4898)
  point P154 (-21.7038, -3.929)
  point P155 (-21.5709, -4.2726)
  point P156 (-21.2483, -4.4055)
  point P157 (-20.9436, -4.3326)
  point P158 (-28.3034, -3.4752)
  point P159 (-28.7767, -3.0036)
  point P160 (-29.2483, -3.4752)
  point P161 (-28.7767, -3.9469)
  point P162 (-3.72, 0.265)
  point P163 (-3.4364, 0.1483)
  point P164 (-4.0198, 0.1467)
  point P165 (-3.6438, -1.1045)
  point P166 (-3.3602, -1.0624)
  point P167 (-3.3391, -0.8176)
  point P168 (-3.647, -0.8841)
  point P169 (-3.271, 0.3056)
  point P170 (-3.7054, 0.4725)
  point P171 (-4.3991, -0.3282)
  point P172 (-7.3796, -0.8727)
  point P173 (-7.6146, -0.7609)
  point P174 (-7.7799, -0.9781)
  point P175 (-7.4461, -1.1126)
  point P176 (-11.3634, 0.3445)
  point P177 (-11.6778, 0.4725)
  point P178 (-12.1365, 0.2132)
  point P179 (-12.5287, 0.4725)
  point P180 (-12.5936, 0.2326)
  point P181 (-12.3829, 0.1273)
  point P182 (-12.0928, 0.0462)
  point P183 (-11.7427, 0.2326)
  point P184 (-11.532, 0.1273)
  point P185 (-17.9112, 0.4725)
  point P186 (-17.9777, 0.2326)
  point P187 (-17.7427, 0.1208)
  point P188 (-19.6778, -0.346)
  point P189 (-19.6244, -0.8792)
  point P190 (-19.9096, -0.6183)
  point P191 (-19.1381, 0.3542)
  point P192 (-19.5903, 0.466)
  point P193 (-19.5919, 0.2423)
  point P194 (-19.3294, 0.1921)
  point P195 (-19.8966, -0.1969)
  point P196 (-20.1705, -0.6361)
  point P197 (-20.0376, -0.9797)
  point P198 (-19.7151, -1.1126)
  point P199 (-19.4104, -1.0397)
  constraints: 1014 other
